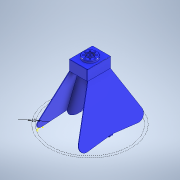
# Autodesk Inventor part: Antena PowerLog
Saved by Autodesk Inventor 2023 (Build 270158000, 158)
## iProperties
Created: 2023-10-25
Part Number: Antena PowerLog
Material: Aluminio 6061
Document SubType Name: Modeling
Designer: jp.reyesf
Density: 2.7 g/cm^3
Appearance: Aluminio - Plano
Author: jp.reyesf
Autodesk Inventor part; units mm, degrees
sketch "Boceto1" plane through (0, 0, 0) normal (0, 1, 0) x (-1, 0, 0)
  line L0 (36.5, 46.5) -> (-36.5, 46.5)
  line L1 (-36.5, 46.5) -> (-36.5, -46.5)
  line L2 (-36.5, -46.5) -> (36.5, -46.5)
  line L3 (36.5, -46.5) -> (36.5, 46.5)
  line L4 (36.5, 46.5) -> (-36.5, -46.5) construction
  line L5 (-36.5, 46.5) -> (36.5, -46.5) construction
  circle A0 centre (0, 0) radius 28
  circle A1 centre (0, 0) radius 15
  circle A2 centre (0, 0) radius 8.5
  line L6 (0, 0) -> (0, 20) construction
  circle A3 centre (0, 20) radius 2.5
  circle A4 centre (0, 0) radius 4
  line L7 (0, 0) -> (-14.1421, 14.1421) construction
  circle A5 centre (-14.1421, 14.1421) radius 2.5
  line L8 (0, 0) -> (-20, 0) construction
  circle A6 centre (-20, 0) radius 2.5
  line L9 (0, 0) -> (-14.1421, -14.1421) construction
  circle A7 centre (-14.1421, -14.1421) radius 2.5
  line L10 (0, 0) -> (0, -20) construction
  circle A8 centre (0, -20) radius 2.5
  line L11 (0, 0) -> (14.1421, -14.1421) construction
  circle A9 centre (14.1421, -14.1421) radius 2.5
  line L12 (0, 0) -> (20, 0) construction
  circle A10 centre (20, 0) radius 2.5
  line L13 (0, 0) -> (14.1421, 14.1421) construction
  circle A11 centre (14.1421, 14.1421) radius 2.5
  dimension "d0" = 93
  dimension "d1" = 73
  dimension "d4" = 56
  dimension "d5" = 30
  dimension "d6" = 17
  dimension "d7" = 20
  dimension "d8" = 5
  dimension "d9" = 8
  dimension "d12" = 360
  constraints: 28 end point, 14 coincident, 12 centre point, 2 midpoint, 2 parallel, 1 horizontal, 1 perpendicular, 1 vertical, 39 other
  measures "d0" distance between parallel lines of L2 L0
  measures "d1" distance between parallel lines of L3 L1
  measures "d4" diameter of A0
  measures "d5" diameter of A1
  measures "d6" diameter of A2
  measures "d7" distance of L6.start L6.end
  measures "d8" diameter of A3
  measures "d9" diameter of A4
extrude "Extrusión1" add sketch "Boceto1" against normal blind 40.5 contours L3 L2 L1 L0 | A0 | A1 | A2 | A3 | A4 | A5 | A6 | A7 | A8 | A9 | A10 | A11
extrude "Extrusión2" add sketch "Boceto1" along normal blind 9 contours A0 | A2
chamfer "Chaflán1" distance 2 angle 45 5 edges at (28, 9, 0) (36.5, -20.25, 46.5) (-36.5, -20.25, 46.5) (36.5, -20.25, -46.5) (-36.5, -20.25, -46.5)
chamfer "Chaflán2" distance 1 angle 45 8 edges at (36.5, 0, 0) (0, 0, -46.5) (35.5, 0, -45.5) (35.5, 0, 45.5) (0, 0, 46.5) (-35.5, 0, 45.5) (-36.5, 0, 0) (-35.5, 0, -45.5)
ref_plane "Plano de trabajo3" through (34.5, -40.5, 0) normal (0, 0, -1) x (-1, 0, 0)
sketch "Boceto2" plane through (34.5, -40.5, 0) normal (0, 0, -1) x (-1, 0, 0)
  line L0 (122, -178.8715) -> (-53, -178.8715)
  line L1 (71, 0) -> (122, -178.8715)
  line L2 (-2, 0) -> (-53, -178.8715)
  point P0 (34.5, 40.5)
  dimension "d23" = 175
  dimension "d24" = 186
  constraints: 6 end point, 2 coincident, 1 equal length, 1 horizontal
  measures "d23" distance of L0.start L0.end
  measures "d24" distance of L1.start L0.start
ref_plane "Plano de trabajo2" through (-36.5, -40.5, -46.5) normal (-0.9616745, 0.2741935, 0) x (0, 0, -1)
sketch "Boceto3" plane through (-36.5, -40.5, -46.5) normal (-0.9616745, 0.2741935, 0) x (0, 0, -1)
  line L0 (-91, 0) -> (-2, 0) projected
  line L1 (-91, 0) -> (-171.9053, 160.7928)
  circle A0 centre (-150.2075, 171.7104) radius 24.2896
  line L2 (-147.7284, 195.8732) -> (-51.5, 186)
  line L3 (-51.5, 186) -> (-41.5, 186)
  line L4 (-41.5, 186) -> (54.7284, 195.8732)
  circle A1 centre (57.2075, 171.7104) radius 24.2896
  line L5 (78.9053, 160.7928) -> (-2, 0)
  line L6 (-46.5, 0) -> (-46.5, 186) projected
  line L7 (-170.5, 158) -> (77.5, 158) construction
  line L8 (-150.2075, 196) -> (57.2075, 196) construction
  point P0 (-46.5, -48.9559)
  point P1 (-46.5, 158)
  dimension "d25" = 248
  dimension "d26" = 158
  dimension "d27" = 10
  dimension "d28" = 180
  dimension "d29" = 10
  constraints: 14 end point, 6 point on circle, 5 tangent, 3 horizontal, 2 centre point, 2 equal length, 2 midpoint, 2 point on line, 1 equal radius
  measures "d25" distance of L7.start L7.end
  measures "d26" distance between parallel lines of L7 L0
  measures "d27" distance of L2.end L3.end
  measures "d28" distance of L0.start L1.end
  measures "d29" distance between parallel lines of L8 L3
extrude "Extrusión3" add sketch "Boceto3" against normal blind 2.25
mirror "Simetría1" about plane through (0, 0, 0) normal (1, 0, 0) of "Extrusión3"
sketch "Boceto4" plane through (34.5, -40.5, 0) normal (0, 0, -1) x (-1, 0, 0)
  line L0 (122, -178.8715) -> (119.8362, -179.4884) projected
  line L1 (122, -178.8715) -> (119.8362, -179.4884) projected
  line L2 (-53, -178.8715) -> (-50.8362, -179.4884) projected
  line L3 (-53, -178.8715) -> (-50.8362, -179.4884) projected
  circle A0 centre (111.1812, -181.9561) radius 9
  line L4 (112.9246, -155.2473) -> (122.5782, -189.1051) projected
  line L5 (0, 0) -> (69, 0) projected
  line L6 (35, 0) -> (34, 0)
  spline S0 degree 3 poles (107.4825, -190.161) (62.0644, -169.6872) (36.3797, -129.0814) (35, 0) knots 0 0 0 0 1 1 1 1
  line L7 (112.9246, -155.2473) -> (68.8362, -0.6169) projected
  line L8 (68.8362, -0.6169) -> (112.9246, -155.2473) projected
  line L9 (112.9246, -155.2473) -> (122.5434, -188.9832) projected
  line L10 (122.5434, -188.9832) -> (119.8362, -179.4884) projected
  line L11 (119.8362, -179.4884) -> (122.5434, -188.9832) projected
  line L12 (122.5434, -188.9832) -> (112.9246, -155.2473) projected
  line L13 (112.9246, -155.2473) -> (68.8362, -0.6169) projected
  line L14 (68.8362, -0.6169) -> (68.6603, 0)
  point P0 (34.5, 40.5)
  point P1 (34.5, 0)
  point P2 (65.5207, -155.8769)
  point P3 (68.8362, -0.6169)
  point P4 (35, 0)
  dimension "d32" = 18
  dimension "d33" = 1
  constraints: 4 end point, 2 midpoint, 2 point on circle, 1 centre point, 1 collinear, 1 horizontal, 1 point on line, 1 tangent, 4 other
  measures "d32" diameter of A0
  measures "d33" distance of L6.start L6.end
extrude "Extrusión4" add sketch "Boceto4" along normal mid plane 10
mirror "Simetría2" about plane through (0, 0, 0) normal (1, 0, 0) of "Extrusión4"
sketch "Boceto5" plane through (0, 9, 0) normal (0, 1, 0) x (1, 0, 0)
  circle A0 centre (0, 0) radius 8.5 projected
  circle A1 centre (0, 0) radius 4 projected
  circle A2 centre (0, 0) radius 15 projected
  circle A3 centre (0, -20) radius 2.5 projected
  circle A4 centre (14.1421, -14.1421) radius 2.5 projected
  circle A5 centre (20, 0) radius 2.5 projected
  circle A6 centre (14.1421, 14.1421) radius 2.5 projected
  circle A7 centre (0, 20) radius 2.5 projected
  circle A8 centre (-14.1421, 14.1421) radius 2.5 projected
  circle A9 centre (-20, 0) radius 2.5 projected
  circle A10 centre (-14.1421, -14.1421) radius 2.5 projected
  circle A11 centre (0, 0) radius 26 projected
  line L0 (-75, 45) -> (25, 45)
  line L1 (25, 45) -> (25, -45)
  line L2 (25, -45) -> (-75, -45)
  line L3 (-75, -45) -> (-75, 45)
  line L4 (25, 0) -> (0, 0) construction
  line L5 (-72, 45) -> (-72, -45)
  dimension "d36" = 25
  dimension "d37" = 100
  dimension "d38" = 3
  dimension "d39" = 90
  constraints: 12 end point, 2 horizontal, 2 parallel, 2 perpendicular, 2 point on line, 1 midpoint
  measures "d36" distance from line of L1 point (0, 0)
  measures "d37" distance between parallel lines of L3 L1
  measures "d38" distance between parallel lines of L5 L3
  measures "d39" distance between parallel lines of L0 L2
extrude "Extrusión5" add sketch "Boceto5" along normal blind 4 separate body contours A0 | A2 | L1 A11 | A11 L1 L2 L5 L0 picked at (-19.8229, 8.0176)
extrude "Extrusión6" add sketch "Boceto5" along normal blind 93 contours L5 L2 L3 L0
fillet "Empalme1" radius 3 2 edges at (-72, 13, 0) (-75, 9, 0)
sketch "Boceto6" plane through (-72, 102, 45) normal (1, 0, 0) x (0, 0, -1)
  line L0 (25, -13.25) -> (25, -68.75) construction
  line L1 (21.75, -13.25) -> (21.75, -68.75)
  line L2 (28.25, -68.75) -> (28.25, -13.25)
  arc A0 (28.25, -13.25) -> (21.75, -13.25) centre (25, -13.25) ccw
  arc A1 (21.75, -68.75) -> (28.25, -68.75) centre (25, -68.75) ccw
  line L3 (65, -13.25) -> (65, -68.75) construction
  line L4 (61.75, -13.25) -> (61.75, -68.75)
  line L5 (68.25, -68.75) -> (68.25, -13.25)
  arc A2 (68.25, -13.25) -> (61.75, -13.25) centre (65, -13.25) ccw
  arc A3 (61.75, -68.75) -> (68.25, -68.75) centre (65, -68.75) ccw
  line L6 (25, -41) -> (65, -41) construction
  line L7 (90, 0) -> (0, 0) projected
  line L8 (45, 0) -> (45, -41) construction
  line L9 (0, -89) -> (90, -89) projected
  point P0 (45, -102)
  dimension "d45" = 40
  dimension "d46" = 6.5
  dimension "d47" = 10
  dimension "d48" = 17
  constraints: 20 end point, 8 point on circle, 8 tangent, 4 centre point, 4 midpoint, 3 parallel, 3 vertical, 1 equal radius, 1 horizontal
  measures "d45" distance of L6.start L6.end
  measures "d46" distance between parallel lines of L1 L2
  measures "d47" distance edge to line of A0 L7
  measures "d48" distance edge to line of A1 L9
extrude "Extrusión7" cut sketch "Boceto6" against normal blind 93
fillet "Empalme2" radius 22 2 edges at (25, 11, 45) (25, 11, -45)
ref_plane "Plano de trabajo4" through (88.0434, -229.4832, -101.2284) normal (0, 1, 0) x (1, 0, 0)
sketch "Boceto7" plane through (0, -229.4832, 0) normal (0, 1, 0) x (1, 0, 0)
  circle A0 centre (0, 0) radius 153.198 construction
  circle A1 centre (0, 0) radius 163.198 construction
  ellipse E0 centre (-83.5819, -103.7075) end of major axis (-83.5819, -79.4179) minor radius 6.6601 (-90.2072, -101.2284) -> (-80.5884, -125.4053) ccw projected
  dimension "d52" = 10
  constraints: 2 centre point, 2 coincident, 2 other
  measures "d52" radial gap between concentric circles of A1 A0
